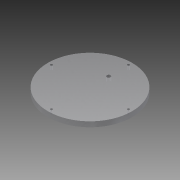
# Autodesk Inventor part: seal3
Saved by Autodesk Inventor 2015 (Build 190159000, 159)
## iProperties
Created: 2015-02-17
Part Number: seal3
Material: Plastic, Transparent
Document SubType Name: Modeling
Designer: Hanjie
Density: 1.188 g/cm^3
Appearance: Transparent - Clear
Author: Hanjie
Autodesk Inventor part; units mm, degrees
ref_plane "YZ Plane" through (0, 0, 0) normal (1, 0, 0) x (0, 1, 0)
ref_plane "XZ Plane" through (0, 0, 0) normal (0, 1, 0) x (-1, 0, 0)
ref_plane "XY Plane" through (0, 0, 0) normal (0, 0, 1) x (1, 0, 0)
sketch "Sketch1" plane through (0, 0, 0) normal (0, 1, 0) x (-1, 0, 0)
  circle A0 centre (0, 0) radius 45.72
  dimension "d0" = 91.44
  constraints: 1 centre point, 1 coincident
  measures "d0" diameter of A0
extrude "Extrusion1" add sketch "Sketch1" along normal blind 5.588
sketch "Sketch2" plane through (0, 5.588, 0) normal (0, 1, 0) x (1, 0, 0)
  circle A0 centre (0, 0) radius 38.1
  line L0 (0, 0) -> (0, 20.32)
  circle A1 centre (0, 20.32) radius 2.032
  line L1 (0, 0) -> (-41.91, 0)
  line L2 (0, 0) -> (0, -41.91)
  line L3 (0, 0) -> (41.91, 0)
  line L4 (0, 0) -> (0, 41.91)
  circle A2 centre (-41.91, 0) radius 1.27
  circle A3 centre (0, 41.91) radius 1.27
  circle A4 centre (41.91, 0) radius 1.27
  circle A5 centre (0, -41.91) radius 1.27
  dimension "d3" = 76.2
  dimension "d4" = 20.32
  dimension "d5" = 4.064
  dimension "d8" = 41.91
  dimension "d9" = 41.91
  dimension "d10" = 41.91
  dimension "d11" = 41.91
  dimension "d12" = 2.54
  dimension "d13" = 2.54
  dimension "d14" = 2.54
  dimension "d15" = 2.54
  constraints: 10 end point, 6 centre point, 6 coincident, 2 horizontal, 2 vertical, 1 point on line
  measures "d3" diameter of A0
  measures "d4" distance of L0.start L0.end
  measures "d5" diameter of A1
  measures "d8" distance of L0.start L1.end
  measures "d9" distance of L0.start L2.end
  measures "d10" distance of L0.start L3.end
  measures "d11" distance of L0.start L4.end
  measures "d12" diameter of A2
  measures "d13" diameter of A3
  measures "d14" diameter of A4
  measures "d15" diameter of A5
extrude "Extrusion2" cut sketch "Sketch2" against normal blind 5.588 contours A5 | A2 | A3 | A4 | L4 L0 A1 | A1 L0 L4
body "Solid1"
